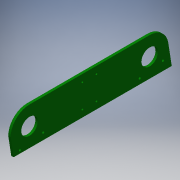
# Autodesk Inventor part: Cross Plate
Saved by Autodesk Inventor 2017 (Build 210142000, 142)
## iProperties
Created: 2017-01-14
Part Number: Cross Plate
Material: Generic
Document SubType Name: Modeling
Designer: Ben
Density: 1 g/cm^3
Appearance: Dark Green
Author: Ben
Autodesk Inventor part; units mm, degrees
ref_plane "YZ Plane" through (0, 0, 0) normal (1, 0, 0) x (0, 1, 0)
ref_plane "XZ Plane" through (0, 0, 0) normal (0, 1, 0) x (-1, 0, 0)
ref_plane "XY Plane" through (0, 0, 0) normal (0, 0, 1) x (1, 0, 0)
sketch "Sketch1" plane through (0, 0, 0) normal (1, 0, 0) x (0, 1, 0)
  line L0 (-50.8, 0) -> (-50.8, -4.023) construction
  line L1 (0, -212.725) -> (0, -187.325) construction
  line L2 (0, 0) -> (-25.4, 0)
  line L3 (0, -212.725) -> (-25.4, -212.725) construction
  line L4 (-25.4, 0) -> (-25.4, -36.5125) construction
  circle A0 centre (-25.4, -25.4) radius 11.1125
  circle A1 centre (-25.4, -187.325) radius 11.1125
  line L5 (0, -106.3625) -> (-50.8, -106.3625) construction
  line L6 (0, -87.3125) -> (-50.8, -87.3125) construction
  line L7 (-50.8, -125.4125) -> (0, -125.4125) construction
  line L8 (-25.4, 0) -> (-50.8, 0) construction
  line L9 (-25.4, -212.725) -> (-50.8, -212.725) construction
  line L10 (-25.4, 0) -> (-50.8, -4.023)
  line L11 (-50.8, -217.0646) -> (-50.8, -212.725)
  line L12 (-50.8, -4.023) -> (-50.8, -212.725)
  line L13 (0, -187.325) -> (0, 0)
  circle A2 centre (-38.5883, -205.4937) radius 1.5875 projected
  circle A3 centre (-43.5687, -174.1367) radius 1.5875 projected
  circle A4 centre (-41.724, -44.0667) radius 1.5875 projected
  circle A5 centre (-46.7044, -12.7098) radius 1.5875 projected
  line L14 (-21.4266, -212.4123) -> (-50.8, -217.0646)
  arc A6 (-21.4266, -212.4123) -> (0, -187.325) centre (-25.4, -187.325) ccw
  line L15 (0, -96.8375) -> (-50.8, -96.8375) construction
  line L16 (0, -115.8875) -> (-50.8, -115.8875) construction
  line L17 (-25.4, -36.5125) -> (-25.4, -176.2125) construction
  line L18 (-25.4, -176.2125) -> (-25.4, -212.725) construction
  line L19 (-9.525, -96.8375) -> (-9.525, -115.8875) construction
  line L20 (-41.275, -96.8375) -> (-41.275, -115.8875) construction
  circle A7 centre (-9.525, -115.8875) radius 1.5875
  circle A8 centre (-9.525, -96.8375) radius 1.5875
  circle A9 centre (-41.275, -115.8875) radius 1.5875
  circle A10 centre (-41.275, -96.8375) radius 1.5875
  point P0 (-25.4, -106.3625)
  dimension "d2" = 22.225
  dimension "d1" = 50.8
  dimension "d3" = 161.925
  dimension "d4" = 25.4
  dimension "d5" = 25.4
  dimension "d10" = 212.725
  dimension "d11" = 38.1
  dimension "d12" = 61.9125
  dimension "d18" = 9
  dimension "d19" = 19.05
  dimension "d20" = 3.175
  dimension "d21" = 31.75
  constraints: 44 end point, 21 point on line, 11 perpendicular, 10 parallel, 5 centre point, 5 coincident, 3 equal radius, 3 vertical, 2 collinear, 2 midpoint, 2 point on circle, 2 tangent, 2 vertical alignment, 7 other
  measures "d1" distance between parallel lines of L1 L0
  measures "d3" distance of point (-25.4, -25.4) point (-25.4, -187.325)
  measures "d4" distance from line of point (-25.4, -187.325) L3
  measures "d5" distance from line of L2 point (-25.4, -25.4)
  measures "d10" distance of L1.start L2.start
  measures "d11" distance between parallel lines of L7 L6
  measures "d12" distance from line of point (-25.4, -187.325) L7
  measures "d18" angle of L9 L14
  measures "d19" distance between parallel lines of L15 L16
  measures "d20" diameter of A7
  measures "d21" distance between parallel lines of L20 L19
extrude "Extrusion1" add sketch "Sketch1" along normal blind 3.175
fillet "Fillet1" radius 25.4 1 edges at (1.5875, 0, 0)
equation "\"d5\" = d4"
body "Solid1"
